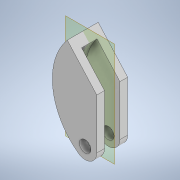
# Autodesk Inventor part: 05-1
Saved by Autodesk Inventor 2022 (Build 260153000, 153)
## iProperties
Created: 2021-09-11
Part Number: 05-1
Material: 일반
Document SubType Name: Modeling
Designer: 서울공업고등학교
Density: 1 g/cm^3
Appearance: 기본값
Author: 서울공업고등학교
Autodesk Inventor part; units mm, degrees
ref_plane "YZ Plane" through (0, 0, 0) normal (1, 0, 0) x (0, 1, 0)
ref_plane "XZ Plane" through (0, 0, 0) normal (0, 1, 0) x (-1, 0, 0)
ref_plane "XY Plane" through (0, 0, 0) normal (0, 0, 1) x (1, 0, 0)
sketch "스케치1" plane through (0, 0, 0) normal (0, 0, 1) x (1, 0, 0)
  line L0 (0, 0) -> (0, -26)
  line L1 (0, 0) -> (26, 0) construction
  arc A0 (-9.5556, -30.833) -> (0, -26) centre (-6, -26) ccw
  line L2 (0, 0) -> (-15.2463, 17)
  arc A1 (-15.2463, 17) -> (-9.5556, -30.833) centre (10, -4.2514) ccw
  circle A2 centre (-6, -26) radius 3
  dimension "d1" = 26
  dimension "d3" = 26
  dimension "d5" = 43
  dimension "d6" = 23
  dimension "d7" = 33
  dimension "d8" = 6
  dimension "d9" = 6
  constraints: 6 end point, 4 point on circle, 3 centre point, 1 coincident, 1 horizontal, 1 perpendicular, 1 tangent, 1 vertical
  measures "d1" distance of L0.start L0.end
  measures "d3" vertical distance of L0.start A0.centre
  measures "d5" vertical distance of A0.centre L2.end
  measures "d6" distance edge to line of A1 L0
  measures "d7" radius of A1
  measures "d8" radius of A0
  measures "d9" diameter of A2
extrude "돌출1" add sketch "스케치1" along normal mid plane 16
ref_plane "작업 평면1" through (0, 0, 0) normal (0, 0, -1) x (-1, 0, 0)
sketch "스케치2" plane through (0, 0, 0) normal (0, 0, -1) x (-1, 0, 0)
  arc A0 (9.5556, -30.833) -> (15.2463, 17) centre (-10, -4.2514) ccw projected
  line L0 (22.8853, -7) -> (17.8648, -7)
  line L1 (0, 0) -> (0, -26) projected
  circle A1 centre (6, -26) radius 3 projected
  arc A2 (17.8648, -7) -> (11.869, 13.2342) centre (-10, -4.2514) ccw
  line L2 (15.2463, 17) -> (0, 0) projected
  arc A3 (0, -26) -> (9.5556, -30.833) centre (6, -26) ccw projected
  dimension "d14" = 19
  constraints: 3 point on circle, 2 end point, 1 centre point, 1 horizontal, 1 point on line
  measures "d14" distance from line of L0 A1.centre
extrude "돌출2" cut sketch "스케치2" along normal mid plane 8 contours A3 L1 L2 A2 L0 A0
